robot2_wedge_lifter_option (Autodesk Fusion 360 design; units mm, degrees)
part number: 2026-09-22-20-04-37-960
part number: 2026-09-22-20-04-48-798
part number: 2026-09-22-20-04-48-802
part number: 2026-09-22-20-04-48-804
part number: 2026-09-22-20-04-48-807
part number: 2026-09-22-20-04-48-809
part number: 2026-09-22-20-10-09-073
part number: 2026-09-22-20-12-27-334
part number: 2026-09-22-20-12-27-362
part number: 2026-09-22-20-14-47-754
part number: 2026-09-22-20-14-47-792
part number: 2026-09-22-20-17-28-654
part number: 2026-09-22-20-20-38-193
part number: 2026-09-22-20-34-57-722
part number: 2026-09-22-20-34-57-795
part number: 2026-09-22-20-34-57-849
part number: 2026-09-22-20-34-57-901
part number: 2026-09-22-20-49-00-878
part number: 2026-09-22-20-49-00-891
part number: 2026-09-22-20-49-00-904
part number: 2026-09-22-20-50-05-757
part number: 2026-09-22-21-16-08-475
part number: 2026-09-22-21-16-09-075
part number: 2026-09-22-21-17-04-467
part number: 2026-09-22-21-17-04-732
part number: 2026-09-22-21-17-05-000
part number: 2026-09-22-21-17-05-645
part number: 2026-09-22-21-40-15-382
part number: 2026-09-22-21-42-45-679
part number: 2026-09-22-22-28-33-537
part number: 2026-09-22-22-50-56-103
part number: 2026-09-22-22-50-56-432
part number: 2026-09-22-22-50-56-745
part number: 2026-09-22-22-50-57-029
part number: 2026-09-22-23-22-03-101
part number: 2026-09-22-23-22-04-161
part number: 2026-09-22-23-22-05-011
part number: 2026-09-22-23-22-05-941
part number: 2026-09-22-23-30-32-609
part number: 2026-09-22-23-30-32-928
part number: 2026-09-22-23-34-46-416
part number: 2026-09-23-02-03-55-828
part number: 2026-09-23-02-03-56-507
part number: 2026-09-23-02-25-34-565
part number: 2026-09-23-02-25-35-125
part number: 2026-09-23-02-25-37-427
part number: 2026-09-23-02-25-38-082
part number: 2026-09-23-02-25-40-527
part number: 2026-09-23-02-25-41-161
part number: 2026-09-23-02-25-43-941
part number: 2026-09-23-02-25-44-578
part number: 2026-09-23-02-25-47-286
part number: 2026-09-23-02-25-47-976
part number: 2026-09-23-02-47-40-033
part number: 2026-09-23-02-47-40-739
part number: 2026-09-23-21-12-34-593
part number: 2026-09-23-21-12-34-998
part number: 2026-09-24-00-47-49-327
part number: 2026-09-24-00-47-50-049
part number: 2026-09-24-00-50-23-317
part number: 2026-09-24-00-50-23-446
part number: 2026-09-24-00-50-24-006
part number: 2026-09-24-00-50-24-800
part number: 2026-09-24-00-50-25-274
part number: 2026-09-24-00-50-26-431
part number: 2026-09-24-00-50-26-900
part number: 2026-09-24-00-50-27-361
part number: 2026-09-24-00-50-27-846
part number: 2026-09-24-00-55-06-014
part number: 2026-09-24-00-55-06-159
part number: 2026-09-24-00-55-06-686
part number: 2026-09-24-00-55-07-196
part number: 2026-09-24-00-55-07-718
part number: 2026-09-24-00-55-08-223
part number: 2026-09-24-00-55-08-760
part number: 2026-09-24-00-55-09-297
part number: 2026-09-24-00-55-09-817
Autodesk Fusion 360 part; units mm, degrees
note: some values were not read from the file. Chosen so that the rebuilt part matches the saved one: which bodies a step acts on.
(part 1 of 3)
sketch "Master_Layout_Top" plane through (0, 0, 0) normal (0, 0, 1) x (1, 0, 0)
  line L0 (80, 90) -> (-80, 90)
  line L1 (-80, 90) -> (-80, -90)
  line L2 (-80, -90) -> (80, -90)
  line L3 (80, -90) -> (80, 90)
  line L4 (0, -90) -> (0, 90) construction
  line L5 (-60.5714, 20.4286) -> (-79.5714, 20.4286)
  line L6 (-79.5714, 20.4286) -> (-79.5714, -21.5714)
  line L7 (-79.5714, -21.5714) -> (-60.5714, -21.5714)
  line L8 (-60.5714, -21.5714) -> (-60.5714, 20.4286)
  line L9 (79.4286, 20.4286) -> (60.4286, 20.4286)
  line L10 (60.4286, 20.4286) -> (60.4286, -21.5714)
  line L11 (60.4286, -21.5714) -> (79.4286, -21.5714)
  line L12 (79.4286, -21.5714) -> (79.4286, 20.4286)
  line L13 (25, -15) -> (-25, -15) construction
  line L14 (-25, -15) -> (-25, -75) construction
  line L15 (-25, -75) -> (25, -75) construction
  line L16 (25, -75) -> (25, -15) construction
  point P0 (0, 90)
  dimension "d14" = 160
  dimension "d15" = 180
  dimension "d16" = 19
  dimension "d17" = 42
  dimension "d18" = 19
  dimension "d19" = 42
  dimension "d20" = 50
  dimension "d21" = 60
  measures "d14" horizontal distance of L0.start L0.end
  measures "d15" vertical distance of L0.end L1.end
  measures "d16" horizontal distance of L5.start L5.end
  measures "d17" vertical distance of L5.end L6.end
  measures "d18" horizontal distance of L9.start L9.end
  measures "d19" vertical distance of L9.end L10.end
  measures "d20" horizontal distance of L13.start L13.end
  measures "d21" vertical distance of L13.end L14.end
sketch "Base_Plate_Sketch" plane through (0, 0, 0) normal (0, 0, 1) x (1, 0, 0) in component "Base_Plate_Al"
  line L0 (80, 90) -> (-80, 90)
  line L1 (-80, 90) -> (-80, -90)
  line L2 (-80, -90) -> (80, -90)
  line L3 (80, -90) -> (80, 90)
  dimension "d26" = 160
  dimension "d27" = 180
  measures "d26" horizontal distance of L0.start L0.end
  measures "d27" vertical distance of L0.end L1.end
extrude "Extrude1" add sketch "Base_Plate_Sketch" against normal blind 2 makes body 1 in component "Base_Plate_Al"
ref_plane "WorkPlane1" through (-80, 0, 0) normal (1, 0, 0) x (0, 1, 0) in component "Left_Side_Plate_Al"
sketch "Left_Plate_Sketch" plane through (-80, 0, 0) normal (1, 0, 0) x (0, 0, -1) in component "Left_Side_Plate_Al"
  line L0 (0, -90) -> (-78, -90)
  line L1 (-78, -90) -> (-78, 90)
  line L2 (-78, 90) -> (0, 90)
  line L3 (0, 90) -> (0, -90)
  dimension "d58" = 78
  dimension "d59" = 180
  measures "d58" horizontal distance of L0.start L0.end
  measures "d59" vertical distance of L0.end L1.end
extrude "Extrude1'" add sketch "Left_Plate_Sketch" along normal blind 2 separate body makes body 2 in component "Left_Side_Plate_Al"
ref_plane "WorkPlane1" through (80, 0, 0) normal (1, 0, 0) x (0, 1, 0) in component "Right_Side_Plate_Al"
sketch "Right_Plate_Sketch" plane through (80, 0, 0) normal (1, 0, 0) x (0, 0, -1) in component "Right_Side_Plate_Al"
  line L0 (0, -90) -> (-78, -90)
  line L1 (-78, -90) -> (-78, 90)
  line L2 (-78, 90) -> (0, 90)
  line L3 (0, 90) -> (0, -90)
  dimension "d64" = 78
  dimension "d65" = 180
  measures "d64" horizontal distance of L0.start L0.end
  measures "d65" vertical distance of L0.end L1.end
extrude "Extrude1''" add sketch "Right_Plate_Sketch" against normal blind 2 separate body makes body 3 in component "Right_Side_Plate_Al"
ref_plane "WorkPlane1" through (-80, 0, 0) normal (1, 0, 0) x (0, 1, 0) in component "Left_Wheel"
sketch "Left_Wheel_Sketch" plane through (-80, 0, 0) normal (1, 0, 0) x (0, 0, -1) in component "Left_Wheel"
  circle A0 centre (-21, 0) radius 21
  dimension "d70" = 42
  dimension "d208" = 21
  measures "d70" diameter of A0
  measures "d208" horizontal distance of origin A0.centre
extrude "Extrude1'''" add sketch "Left_Wheel_Sketch" along normal blind 19 separate body makes body 4 in component "Left_Wheel"
ref_plane "WorkPlane1" through (80, 0, 0) normal (1, 0, 0) x (0, 1, 0) in component "Right_Wheel"
sketch "Right_Wheel_Sketch" plane through (80, 0, 0) normal (1, 0, 0) x (0, 0, -1) in component "Right_Wheel"
  circle A0 centre (-21, 0) radius 21
  dimension "d75" = 42
  dimension "d209" = 21
  measures "d75" diameter of A0
  measures "d209" horizontal distance of origin A0.centre
extrude "Extrude1''''" add sketch "Right_Wheel_Sketch" against normal blind 19 separate body makes body 5 in component "Right_Wheel"
ref_plane "WorkPlane1" through (0, 0, 78) normal (0, 0, 1) x (1, 0, 0) in component "Top_Cover"
sketch "Top_Cover_Sketch" plane through (0, 0, 78) normal (0, 0, 1) x (1, 0, 0) in component "Top_Cover"
  line L0 (80, 90) -> (-80, 90)
  line L1 (-80, 90) -> (-80, -90)
  line L2 (-80, -90) -> (80, -90)
  line L3 (80, -90) -> (80, 90)
  dimension "d106" = 160
  dimension "d107" = 180
  measures "d106" horizontal distance of L0.start L0.end
  measures "d107" vertical distance of L0.end L1.end
extrude "Extrude1'''''" add sketch "Top_Cover_Sketch" along normal blind 2 separate body makes body 6 in component "Top_Cover"
sketch "Left_WedgeTrim_Sketch" plane through (-80, 0, 0) normal (1, 0, 0) x (0, 0, -1) in component "Left_Side_Plate_Al"
  line L0 (100, 40) -> (-100, 40)
  line L1 (-100, 40) -> (-100, 92)
  line L2 (-100, 92) -> (100, 92)
  line L3 (100, 92) -> (100, 40)
extrude "Extrude4" cut sketch "Left_WedgeTrim_Sketch" along normal mid plane 10 bodies 2 in component "Left_Side_Plate_Al"
sketch "Right_WedgeTrim_Sketch" plane through (80, 0, 0) normal (1, 0, 0) x (0, 0, -1) in component "Right_Side_Plate_Al"
  line L0 (100, 40) -> (-100, 40)
  line L1 (-100, 40) -> (-100, 92)
  line L2 (-100, 92) -> (100, 92)
  line L3 (100, 92) -> (100, 40)
extrude "Extrude4'" cut sketch "Right_WedgeTrim_Sketch" along normal mid plane 10 bodies 3 in component "Right_Side_Plate_Al"
sketch "Left_WheelWell_Sketch" plane through (-80, 0, 0) normal (1, 0, 0) x (0, 0, -1) in component "Left_Side_Plate_Al"
  line L0 (10, -26) -> (-42, -26)
  line L1 (-42, -26) -> (-42, 26)
  line L2 (-42, 26) -> (10, 26)
  line L3 (10, 26) -> (10, -26)
extrude "Extrude5" cut sketch "Left_WheelWell_Sketch" along normal mid plane 10 bodies 2 in component "Left_Side_Plate_Al"
sketch "Right_WheelWell_Sketch" plane through (80, 0, 0) normal (1, 0, 0) x (0, 0, -1) in component "Right_Side_Plate_Al"
  line L0 (10, -26) -> (-42, -26)
  line L1 (-42, -26) -> (-42, 26)
  line L2 (-42, 26) -> (10, 26)
  line L3 (10, 26) -> (10, -26)
extrude "Extrude5'" cut sketch "Right_WheelWell_Sketch" along normal mid plane 10 bodies 3 in component "Right_Side_Plate_Al"
ref_plane "WorkPlane1" through (-61, 0, 0) normal (1, 0, 0) x (0, 1, 0) in component "TT_Gearbox_L"
sketch "TT_Gearbox_L_Sketch" plane through (-61, 0, 0) normal (1, 0, 0) x (0, 0, -1) in component "TT_Gearbox_L"
  line L0 (-12, 11) -> (-30, 11)
  line L1 (-30, 11) -> (-30, -11)
  line L2 (-30, -11) -> (-12, -11)
  line L3 (-12, -11) -> (-12, 11)
  dimension "d228" = 18
  dimension "d229" = 22
  measures "d228" horizontal distance of L0.start L0.end
  measures "d229" vertical distance of L0.end L1.end
extrude "Extrude1''''''" add sketch "TT_Gearbox_L_Sketch" along normal blind 24 separate body makes body 7 in component "TT_Gearbox_L"
ref_plane "WorkPlane1" through (-3.7, 0, 0) normal (1, 0, 0) x (0, 1, 0) in component "TT_Motor_Can_L"
sketch "TT_Motor_Can_L_Sketch" plane through (-3.7, 0, 0) normal (1, 0, 0) x (0, 0, -1) in component "TT_Motor_Can_L"
  circle A0 centre (-21, 0) radius 10
  dimension "d234" = 20
  measures "d234" diameter of A0
extrude "Extrude2" add sketch "TT_Motor_Can_L_Sketch" against normal blind 25 separate body makes body 8 in component "TT_Motor_Can_L"
ref_plane "WorkPlane1" through (61, 0, 0) normal (1, 0, 0) x (0, 1, 0) in component "TT_Gearbox_R"
sketch "TT_Gearbox_R_Sketch" plane through (61, 0, 0) normal (1, 0, 0) x (0, 0, -1) in component "TT_Gearbox_R"
  line L0 (-12, 11) -> (-30, 11)
  line L1 (-30, 11) -> (-30, -11)
  line L2 (-30, -11) -> (-12, -11)
  line L3 (-12, -11) -> (-12, 11)
  dimension "d241" = 18
  dimension "d242" = 22
  measures "d241" horizontal distance of L0.start L0.end
  measures "d242" vertical distance of L0.end L1.end
extrude "Extrude1'''''''" add sketch "TT_Gearbox_R_Sketch" against normal blind 24 separate body makes body 9 in component "TT_Gearbox_R"
ref_plane "WorkPlane1" through (3.7, 0, 0) normal (1, 0, 0) x (0, 1, 0) in component "TT_Motor_Can_R"
sketch "TT_Motor_Can_R_Sketch" plane through (3.7, 0, 0) normal (1, 0, 0) x (0, 0, -1) in component "TT_Motor_Can_R"
  circle A0 centre (-21, 0) radius 10
  dimension "d247" = 20
  measures "d247" diameter of A0
extrude "Extrude2'" add sketch "TT_Motor_Can_R_Sketch" along normal blind 25 separate body makes body 10 in component "TT_Motor_Can_R"
ref_plane "WorkPlane1" through (0, 0, 31.6) normal (0, 0, 1) x (1, 0, 0) in component "Battery_and_Tray"
sketch "Battery_and_Tray_Sketch" plane through (0, 0, 31.6) normal (0, 0, 1) x (1, 0, 0) in component "Battery_and_Tray"
  line L0 (-52, -55.5) -> (52, -55.5)
  line L1 (52, -55.5) -> (52, -20.5)
  line L2 (52, -20.5) -> (-52, -20.5)
  line L3 (-52, -20.5) -> (-52, -55.5)
  dimension "d430" = 104
  dimension "d431" = 35
  measures "d430" horizontal distance of L0.start L0.end
  measures "d431" vertical distance of L0.end L1.end
extrude "Extrude1''''''''" add sketch "Battery_and_Tray_Sketch" along normal blind 27 separate body makes body 11 in component "Battery_and_Tray"
sketch "Left_Base_WheelCut_Sketch" plane through (0, 0, 0) normal (0, 0, 1) x (1, 0, 0) in component "Base_Plate_Al"
  line L0 (-90, -24) -> (-58, -24)
  line L1 (-58, -24) -> (-58, 24)
  line L2 (-58, 24) -> (-90, 24)
  line L3 (-90, 24) -> (-90, -24)
extrude "Extrude2''" cut sketch "Left_Base_WheelCut_Sketch" along normal mid plane 10 bodies 1 in component "Base_Plate_Al"
sketch "Right_Base_WheelCut_Sketch" plane through (0, 0, 0) normal (0, 0, 1) x (1, 0, 0) in component "Base_Plate_Al"
  line L0 (90, -24) -> (58, -24)
  line L1 (58, -24) -> (58, 24)
  line L2 (58, 24) -> (90, 24)
  line L3 (90, 24) -> (90, -24)
extrude "Extrude3" cut sketch "Right_Base_WheelCut_Sketch" along normal mid plane 10 bodies 1 in component "Base_Plate_Al"
move_body "GroundClearanceOffset" bodies 1 to x (1, 0, 0) y (0, 1, 0) z (0, 0, 1) at (0, 0, 5) in component "Base_Plate_Al"
move_body "GroundClearanceOffset'" bodies 2 to x (1, 0, 0) y (0, 1, 0) z (0, 0, 1) at (0, 0, 5) in component "Left_Side_Plate_Al"
move_body "GroundClearanceOffset''" bodies 3 to x (1, 0, 0) y (0, 1, 0) z (0, 0, 1) at (0, 0, 5) in component "Right_Side_Plate_Al"
move_body "GroundClearanceOffset'''" bodies 6 to x (1, 0, 0) y (0, 1, 0) z (0, 0, 1) at (0, 0, 5) in component "Top_Cover"
ref_plane "WorkPlane1" through (-80, 0, 0) normal (1, 0, 0) x (0, 1, 0) in component "Front_Wedge_L"
sketch "L_Wedge_Sketch" plane through (-80, 0, 0) normal (1, 0, 0) x (0, 0, -1) in component "Front_Wedge_L"
  line L0 (0, 90) -> (0, 40)
  line L1 (0, 40) -> (-78, 40)
  line L2 (-78, 40) -> (0, 90)
  dimension "d488" = 50
  dimension "d489" = 78
  dimension "d490" = 90
  measures "d488" vertical distance of L0.start L0.end
  measures "d489" horizontal distance of L0.end L1.end
  measures "d490" vertical distance of origin L0.start
extrude "Extrude1'''''''''" add sketch "L_Wedge_Sketch" along normal blind 45 separate body makes body 12 in component "Front_Wedge_L"
move_body "Move1" bodies 12 to x (1, 0, 0) y (0, 1, 0) z (0, 0, 1) at (0, 0, 5) in component "Front_Wedge_L"
ref_plane "WorkPlane1" through (80, 0, 0) normal (1, 0, 0) x (0, 1, 0) in component "Front_Wedge_R"
sketch "R_Wedge_Sketch" plane through (80, 0, 0) normal (1, 0, 0) x (0, 0, -1) in component "Front_Wedge_R"
  line L0 (0, 90) -> (0, 40)
  line L1 (0, 40) -> (-78, 40)
  line L2 (-78, 40) -> (0, 90)
  dimension "d498" = 50
  dimension "d499" = 78
  dimension "d500" = 90
  measures "d498" vertical distance of L0.start L0.end
  measures "d499" horizontal distance of L0.end L1.end
  measures "d500" vertical distance of origin L0.start
extrude "Extrude1''''''''''" add sketch "R_Wedge_Sketch" against normal blind 45 separate body makes body 13 in component "Front_Wedge_R"
move_body "Move1'" bodies 13 to x (1, 0, 0) y (0, 1, 0) z (0, 0, 1) at (0, 0, 5) in component "Front_Wedge_R"
ref_plane "WorkPlane1" through (-32.5, 0, 0) normal (1, 0, 0) x (0, 1, 0) in component "Spinner_Shaft"
sketch "Spinner_Shaft_Sketch" plane through (-32.5, 0, 0) normal (1, 0, 0) x (0, 0, -1) in component "Spinner_Shaft"
  circle A0 centre (-38.5, 75) radius 2
  dimension "d508" = 4
  measures "d508" diameter of A0
extrude "Extrude1'''''''''''" add sketch "Spinner_Shaft_Sketch" along normal blind 65 separate body makes body 14 in component "Spinner_Shaft"
ref_plane "WorkPlane1" through (-32.5, 0, 0) normal (1, 0, 0) x (0, 1, 0) in component "Left_Support"
sketch "Left_Support_Sketch" plane through (-32.5, 0, 0) normal (1, 0, 0) x (0, 0, -1) in component "Left_Support"
  circle A0 centre (-38.5, 75) radius 6.5
  dimension "d513" = 13
  measures "d513" diameter of A0
extrude "Extrude1''''''''''''" add sketch "Left_Support_Sketch" along normal blind 10 separate body makes body 15 in component "Left_Support"
ref_plane "WorkPlane1" through (32.5, 0, 0) normal (1, 0, 0) x (0, 1, 0) in component "Right_Support"
sketch "Right_Support_Sketch" plane through (32.5, 0, 0) normal (1, 0, 0) x (0, 0, -1) in component "Right_Support"
  circle A0 centre (-38.5, 75) radius 6.5
  dimension "d518" = 13
  measures "d518" diameter of A0
extrude "Extrude1'''''''''''''" add sketch "Right_Support_Sketch" against normal blind 10 separate body makes body 16 in component "Right_Support"
ref_plane "WorkPlane1" through (-15, 0, 0) normal (1, 0, 0) x (0, 1, 0) in component "Spinner_Motor"
sketch "Spinner_Motor_Sketch" plane through (-15, 0, 0) normal (1, 0, 0) x (0, 0, -1) in component "Spinner_Motor"
  circle A0 centre (-38.5, 25.75) radius 13.75
  dimension "d528" = 27.5
  measures "d528" diameter of A0
extrude "Extrude1''''''''''''''" add sketch "Spinner_Motor_Sketch" along normal blind 30 separate body makes body 17 in component "Spinner_Motor"
sketch "Standoff_Base_Sketch" plane through (0, 0, 0) normal (0, 0, 1) x (1, 0, 0) in component "Standoffs_Fasteners"
  circle A0 centre (-75, -85) radius 3
  circle A1 centre (-75, -85) radius 1.6
  circle A2 centre (75, -85) radius 3
  circle A3 centre (75, -85) radius 1.6
  circle A4 centre (-75, 35) radius 3
  circle A5 centre (-75, 35) radius 1.6
  circle A6 centre (75, 35) radius 3
  circle A7 centre (75, 35) radius 1.6
  dimension "d563" = 6
  dimension "d564" = 3.2
  dimension "d565" = 6
  dimension "d566" = 3.2
  dimension "d567" = 6
  dimension "d568" = 3.2
  dimension "d569" = 6
  dimension "d570" = 3.2
  measures "d563" diameter of A0
  measures "d564" diameter of A1
  measures "d565" diameter of A2
  measures "d566" diameter of A3
  measures "d567" diameter of A4
  measures "d568" diameter of A5
  measures "d569" diameter of A6
  measures "d570" diameter of A7
extrude "Extrude1'''''''''''''''" add sketch "Standoff_Base_Sketch" along normal blind 78 from surface at 5 separate body contours A0 | A1 | A2 | A3 | A4 | A5 | A6 | A7 makes body 18 at (-76.3686, 32.3304, 31) makes body 19 at (72.3653, -86.4348, 57) makes body 20 at (-77.6347, -86.4348, 57) makes body 21 at (73.6314, 32.3304, 31) in component "Standoffs_Fasteners"
sketch "Base_Plate_Al_FastenerHoles" plane through (0, 0, 0) normal (0, 0, 1) x (1, 0, 0) in component "Base_Plate_Al"
  circle A0 centre (-75, -85) radius 1.7
  circle A1 centre (75, -85) radius 1.7
  circle A2 centre (-75, 35) radius 1.7
  circle A3 centre (75, 35) radius 1.7
extrude "Extrude4''" cut sketch "Base_Plate_Al_FastenerHoles" along normal mid plane 8 bodies 1 in component "Base_Plate_Al"
sketch "Top_Cover_FastenerHoles" plane through (0, 0, 0) normal (0, 0, 1) x (1, 0, 0) in component "Top_Cover"
  circle A0 centre (-75, -85) radius 1.7
  circle A1 centre (75, -85) radius 1.7
  circle A2 centre (-75, 35) radius 1.7
  circle A3 centre (75, 35) radius 1.7
extrude "Extrude2'''" cut sketch "Top_Cover_FastenerHoles" along normal mid plane 8 bodies 6 in component "Top_Cover"
sketch "Left_FastenerHoles_Sketch" plane through (-80, 0, 0) normal (1, 0, 0) x (0, 0, -1) in component "Left_Side_Plate_Al"
  circle A0 centre (-44, -85) radius 1.7
  circle A1 centre (-44, 35) radius 1.7
extrude "Extrude6" cut sketch "Left_FastenerHoles_Sketch" along normal mid plane 10 bodies 2 in component "Left_Side_Plate_Al"
sketch "Right_FastenerHoles_Sketch" plane through (80, 0, 0) normal (1, 0, 0) x (0, 0, -1) in component "Right_Side_Plate_Al"
  circle A0 centre (-44, -85) radius 1.7
  circle A1 centre (-44, 35) radius 1.7
extrude "Extrude6'" cut sketch "Right_FastenerHoles_Sketch" along normal mid plane 10 bodies 3 in component "Right_Side_Plate_Al"
sketch "L_TT_MountHoles" plane through (-61, 0, 0) normal (1, 0, 0) x (0, 0, -1) in component "TT_Gearbox_L"
  circle A0 centre (-21, -8.75) radius 1.7
  circle A1 centre (-21, 8.75) radius 1.7
extrude "Extrude2''''" cut sketch "L_TT_MountHoles" along normal mid plane 72 bodies 7 in component "TT_Gearbox_L"
sketch "R_TT_MountHoles" plane through (61, 0, 0) normal (1, 0, 0) x (0, 0, -1) in component "TT_Gearbox_R"
  circle A0 centre (-21, -8.75) radius 1.7
  circle A1 centre (-21, 8.75) radius 1.7
extrude "Extrude2'''''" cut sketch "R_TT_MountHoles" along normal mid plane 72 bodies 9 in component "TT_Gearbox_R"
sketch "Spinner_Motor_MountHoles" plane through (-15, 0, 0) normal (1, 0, 0) x (0, 0, -1) in component "Spinner_Motor"
  circle A0 centre (-8, -9.5) radius 1.7
  circle A1 centre (-8, 9.5) radius 1.7
  circle A2 centre (8, -9.5) radius 1.7
  circle A3 centre (8, 9.5) radius 1.7
extrude "Extrude2''''''" cut sketch "Spinner_Motor_MountHoles" along normal mid plane 90 bodies 17 in component "Spinner_Motor"
sketch "Servo_FlangeHoles" plane through (0, 0, 0) normal (0, 0, 1) x (1, 0, 0) in component "Top_Cover"
  circle A0 centre (0, -24.75) radius 1.7
  circle A1 centre (0, 24.75) radius 1.7
extrude "Extrude3'" cut sketch "Servo_FlangeHoles" along normal mid plane 8 bodies 6 in component "Top_Cover"
ref_plane "WorkPlane1" through (0, 0, 29.6) normal (0, 0, 1) x (1, 0, 0) in component "Battery_Holder"
sketch "Holder_Floor_Sketch" plane through (0, 0, 29.6) normal (0, 0, 1) x (1, 0, 0) in component "Battery_Holder"
  line L0 (-52, -55.5) -> (52, -55.5)
  line L1 (52, -55.5) -> (52, -20.5)
  line L2 (52, -20.5) -> (-52, -20.5)
  line L3 (-52, -20.5) -> (-52, -55.5)
  dimension "d597" = 104
  dimension "d598" = 35
  measures "d597" horizontal distance of L0.start L0.end
  measures "d598" vertical distance of L0.end L1.end
extrude "Extrude1''''''''''''''''" add sketch "Holder_Floor_Sketch" along normal blind 2 separate body makes body 22 in component "Battery_Holder"
sketch "Holder_StrapSlots" plane through (0, 0, 29.6) normal (0, 0, 1) x (1, 0, 0) in component "Battery_Holder"
  line L0 (-39, -43) -> (-35, -43)
  line L1 (-35, -43) -> (-35, -33)
  line L2 (-35, -33) -> (-39, -33)
  line L3 (-39, -33) -> (-39, -43)
  line L4 (35, -43) -> (39, -43)
  line L5 (39, -43) -> (39, -33)
  line L6 (39, -33) -> (35, -33)
  line L7 (35, -33) -> (35, -43)
extrude "Extrude2'''''''" cut sketch "Holder_StrapSlots" along normal mid plane 10 bodies 22 in component "Battery_Holder"
ref_plane "WorkPlane2" through (0, 0, 31.6) normal (0, 0, 1) x (1, 0, 0) in component "Battery_Holder"
sketch "Sketch3" plane through (0, 0, 31.6) normal (0, 0, 1) x (1, 0, 0) in component "Battery_Holder"
  line L0 (-52, -57.5) -> (52, -57.5)
  line L1 (52, -57.5) -> (52, -55.5)
  line L2 (52, -55.5) -> (-52, -55.5)
  line L3 (-52, -55.5) -> (-52, -57.5)
extrude "Extrude3''" add sketch "Sketch3" along normal blind 5 bodies 22 in component "Battery_Holder"
sketch "Sketch4" plane through (0, 0, 31.6) normal (0, 0, 1) x (1, 0, 0) in component "Battery_Holder"
  line L0 (-52, -20.5) -> (52, -20.5)
  line L1 (52, -20.5) -> (52, -18.5)
  line L2 (52, -18.5) -> (-52, -18.5)
  line L3 (-52, -18.5) -> (-52, -20.5)
extrude "Extrude4'''" add sketch "Sketch4" along normal blind 5 bodies 22 in component "Battery_Holder"
move_body "Move1''" bodies 22 to x (1, 0, 0) y (0, 1, 0) z (0, 0, 1) at (0, 0, 3) in component "Battery_Holder"
move_body "Move1'''" bodies 11 to x (1, 0, 0) y (0, 1, 0) z (0, 0, 1) at (0, 0, 3) in component "Battery_and_Tray"
sketch "L_Wedge_ScrewHoles" plane through (0, 0, 0) normal (0, 0, 1) x (1, 0, 0) in component "Front_Wedge_L"
  circle A0 centre (-73, 80) radius 1.7
  circle A1 centre (-50, 50) radius 1.7
extrude "Extrude2''''''''" cut sketch "L_Wedge_ScrewHoles" along normal mid plane 12 bodies 12 in component "Front_Wedge_L"
sketch "L_WedgeScrew_BaseHoles" plane through (0, 0, 0) normal (0, 0, 1) x (1, 0, 0) in component "Base_Plate_Al"
  circle A0 centre (-73, 80) radius 1.7
  circle A1 centre (-50, 50) radius 1.7
extrude "Extrude6''" cut sketch "L_WedgeScrew_BaseHoles" along normal mid plane 12 bodies 1 in component "Base_Plate_Al"
sketch "R_Wedge_ScrewHoles" plane through (0, 0, 0) normal (0, 0, 1) x (1, 0, 0) in component "Front_Wedge_R"
  circle A0 centre (73, 80) radius 1.7
  circle A1 centre (50, 50) radius 1.7
extrude "Extrude2'''''''''" cut sketch "R_Wedge_ScrewHoles" along normal mid plane 12 bodies 13 in component "Front_Wedge_R"
sketch "R_WedgeScrew_BaseHoles" plane through (0, 0, 0) normal (0, 0, 1) x (1, 0, 0) in component "Base_Plate_Al"
  circle A0 centre (73, 80) radius 1.7
  circle A1 centre (50, 50) radius 1.7
extrude "Extrude7" cut sketch "R_WedgeScrew_BaseHoles" along normal mid plane 12 bodies 1 in component "Base_Plate_Al"
sketch "Left_TT_MountHoles" plane through (-80, 0, 0) normal (1, 0, 0) x (0, 0, -1) in component "Left_Side_Plate_Al"
  circle A0 centre (-21, -8.75) radius 1.7
  circle A1 centre (-21, 8.75) radius 1.7
extrude "Extrude7'" cut sketch "Left_TT_MountHoles" along normal mid plane 12 bodies 2 in component "Left_Side_Plate_Al"
sketch "Right_TT_MountHoles" plane through (80, 0, 0) normal (1, 0, 0) x (0, 0, -1) in component "Right_Side_Plate_Al"
  circle A0 centre (-21, -8.75) radius 1.7
  circle A1 centre (-21, 8.75) radius 1.7
extrude "Extrude7''" cut sketch "Right_TT_MountHoles" along normal mid plane 12 bodies 3 in component "Right_Side_Plate_Al"
sketch "RollPin_Hole" plane through (0, 0, 0) normal (0, 0, 1) x (1, 0, 0) in component "Spinner_Shaft"
  circle A0 centre (0, 75) radius 1
extrude "Extrude2''''''''''" cut sketch "RollPin_Hole" along normal mid plane 60 bodies 14 in component "Spinner_Shaft"
sketch "Cradle_Block_Sketch" plane through (0, 0, 0) normal (0, 0, 1) x (1, 0, 0) in component "Spinner_Motor_Cradle"
  line L0 (-15, 12) -> (15, 12)
  line L1 (15, 12) -> (15, 41)
  line L2 (15, 41) -> (-15, 41)
  line L3 (-15, 41) -> (-15, 12)
extrude "Extrude1'''''''''''''''''" add sketch "Cradle_Block_Sketch" along normal blind 25.5 from surface at 5 separate body makes body 23 in component "Spinner_Motor_Cradle"
sketch "Cradle_Saddle_Sketch" plane through (0, 0, 0) normal (1, 0, 0) x (0, 0, -1) in component "Spinner_Motor_Cradle"
  circle A0 centre (-38.5, 25.75) radius 14.15
extrude "Extrude2'''''''''''" cut sketch "Cradle_Saddle_Sketch" along normal mid plane 50 bodies 23 in component "Spinner_Motor_Cradle"
sketch "Cradle_Bolt_Sketch" plane through (0, 0, 0) normal (0, 0, 1) x (1, 0, 0) in component "Spinner_Motor_Cradle"
  circle A0 centre (-11, 16) radius 1.25
  circle A1 centre (11, 16) radius 1.25
  circle A2 centre (-11, 37) radius 1.25
  circle A3 centre (11, 37) radius 1.25
extrude "Extrude3'''" cut sketch "Cradle_Bolt_Sketch" along normal blind 8 from surface at 5 bodies 23 in component "Spinner_Motor_Cradle"
sketch "Cradle_Bolt_Clearance_Sketch" plane through (0, 0, 0) normal (0, 0, 1) x (1, 0, 0) in component "Base_Plate_Al"
  circle A0 centre (-11, 16) radius 1.7
  circle A1 centre (11, 16) radius 1.7
  circle A2 centre (-11, 37) radius 1.7
  circle A3 centre (11, 37) radius 1.7
extrude "Extrude8" cut sketch "Cradle_Bolt_Clearance_Sketch" along normal mid plane 30 bodies 1 in component "Base_Plate_Al"
sketch "TT_Mount_Clearance_Sketch_L" plane through (0, 0, 0) normal (0, 0, 1) x (1, 0, 0) in component "Base_Plate_Al"
  circle A0 centre (-51, -14) radius 1.7
  circle A1 centre (-51, 14) radius 1.7
  circle A2 centre (-38.7, -14) radius 1.7
  circle A3 centre (-38.7, 14) radius 1.7
extrude "Extrude10" cut sketch "TT_Mount_Clearance_Sketch_L" along normal mid plane 30 bodies 1 in component "Base_Plate_Al"
sketch "TT_Mount_Clearance_Sketch_R" plane through (0, 0, 0) normal (0, 0, 1) x (1, 0, 0) in component "Base_Plate_Al"
  circle A0 centre (38.7, -14) radius 1.7
  circle A1 centre (38.7, 14) radius 1.7
  circle A2 centre (51, -14) radius 1.7
  circle A3 centre (51, 14) radius 1.7
extrude "Extrude11" cut sketch "TT_Mount_Clearance_Sketch_R" along normal mid plane 30 bodies 1 in component "Base_Plate_Al"
sketch "TT_Mount_Block_Sketch" plane through (0, 0, 0) normal (0, 0, 1) x (1, 0, 0) in component "TT_Motor_Mount_L"
  line L0 (-55, -16.5) -> (-34.7, -16.5)
  line L1 (-34.7, -16.5) -> (-34.7, 16.5)
  line L2 (-34.7, 16.5) -> (-55, 16.5)
  line L3 (-55, 16.5) -> (-55, -16.5)
extrude "Extrude1''''''''''''''''''" add sketch "TT_Mount_Block_Sketch" along normal blind 23.5 from surface at 5 separate body makes body 24 in component "TT_Motor_Mount_L"
sketch "TT_Mount_Pocket_Sketch" plane through (0, 0, 0) normal (0, 0, 1) x (1, 0, 0) in component "TT_Motor_Mount_L"
  line L0 (-60, -11.5) -> (-29.7, -11.5)
  line L1 (-29.7, -11.5) -> (-29.7, 11.5)
  line L2 (-29.7, 11.5) -> (-60, 11.5)
  line L3 (-60, 11.5) -> (-60, -11.5)
extrude "Extrude2''''''''''''" cut sketch "TT_Mount_Pocket_Sketch" along normal blind 26.5 from surface at 12 bodies 24 in component "TT_Motor_Mount_L"
sketch "TT_Mount_Bolt_Sketch" plane through (0, 0, 0) normal (0, 0, 1) x (1, 0, 0) in component "TT_Motor_Mount_L"
  circle A0 centre (-51, -14) radius 1.25
  circle A1 centre (-51, 14) radius 1.25
  circle A2 centre (-38.7, -14) radius 1.25
  circle A3 centre (-38.7, 14) radius 1.25
extrude "Extrude3''''" cut sketch "TT_Mount_Bolt_Sketch" along normal blind 5 from surface at 5 bodies 24 in component "TT_Motor_Mount_L"
sketch "TT_Mount_ClampTap_Sketch" plane through (0, 0, 0) normal (0, 0, 1) x (1, 0, 0) in component "TT_Motor_Mount_L"
  circle A0 centre (-44.85, -14) radius 1.25
  circle A1 centre (-44.85, 14) radius 1.25
extrude "Extrude4''''" cut sketch "TT_Mount_ClampTap_Sketch" against normal blind 8 from surface at 28.5 bodies 24 in component "TT_Motor_Mount_L"
sketch "TT_Clamp_Sketch" plane through (0, 0, 0) normal (0, 0, 1) x (1, 0, 0) in component "TT_Motor_Clamp_L"
  line L0 (-49.85, -16.5) -> (-39.85, -16.5)
  line L1 (-39.85, -16.5) -> (-39.85, 16.5)
  line L2 (-39.85, 16.5) -> (-49.85, 16.5)
  line L3 (-49.85, 16.5) -> (-49.85, -16.5)
extrude "Extrude1'''''''''''''''''''" add sketch "TT_Clamp_Sketch" along normal blind 3 from surface at 30 separate body makes body 25 in component "TT_Motor_Clamp_L"
sketch "TT_Clamp_Holes_Sketch" plane through (0, 0, 0) normal (0, 0, 1) x (1, 0, 0) in component "TT_Motor_Clamp_L"
  circle A0 centre (-44.85, -14) radius 1.7
  circle A1 centre (-44.85, 14) radius 1.7
extrude "Extrude2'''''''''''''" cut sketch "TT_Clamp_Holes_Sketch" along normal mid plane 200 bodies 25 in component "TT_Motor_Clamp_L"
sketch "TT_Mount_Block_Sketch (2)" plane through (0, 0, 0) normal (0, 0, 1) x (1, 0, 0) in component "TT_Motor_Mount_R"
  line L0 (34.7, -16.5) -> (55, -16.5)
  line L1 (55, -16.5) -> (55, 16.5)
  line L2 (55, 16.5) -> (34.7, 16.5)
  line L3 (34.7, 16.5) -> (34.7, -16.5)
extrude "Extrude1''''''''''''''''''''" add sketch "TT_Mount_Block_Sketch (2)" along normal blind 23.5 from surface at 5 separate body makes body 26 in component "TT_Motor_Mount_R"
sketch "TT_Mount_Pocket_Sketch (2)" plane through (0, 0, 0) normal (0, 0, 1) x (1, 0, 0) in component "TT_Motor_Mount_R"
  line L0 (29.7, -11.5) -> (60, -11.5)
  line L1 (60, -11.5) -> (60, 11.5)
  line L2 (60, 11.5) -> (29.7, 11.5)
  line L3 (29.7, 11.5) -> (29.7, -11.5)
extrude "Extrude2''''''''''''''" cut sketch "TT_Mount_Pocket_Sketch (2)" along normal blind 26.5 from surface at 12 bodies 26 in component "TT_Motor_Mount_R"
sketch "TT_Mount_Bolt_Sketch (2)" plane through (0, 0, 0) normal (0, 0, 1) x (1, 0, 0) in component "TT_Motor_Mount_R"
  circle A0 centre (38.7, -14) radius 1.25
  circle A1 centre (38.7, 14) radius 1.25
  circle A2 centre (51, -14) radius 1.25
  circle A3 centre (51, 14) radius 1.25
extrude "Extrude3'''''" cut sketch "TT_Mount_Bolt_Sketch (2)" along normal blind 5 from surface at 5 bodies 26 in component "TT_Motor_Mount_R"
sketch "TT_Mount_ClampTap_Sketch (2)" plane through (0, 0, 0) normal (0, 0, 1) x (1, 0, 0) in component "TT_Motor_Mount_R"
  circle A0 centre (44.85, -14) radius 1.25
  circle A1 centre (44.85, 14) radius 1.25
extrude "Extrude4'''''" cut sketch "TT_Mount_ClampTap_Sketch (2)" against normal blind 8 from surface at 28.5 bodies 26 in component "TT_Motor_Mount_R"
sketch "TT_Clamp_Sketch (2)" plane through (0, 0, 0) normal (0, 0, 1) x (1, 0, 0) in component "TT_Motor_Clamp_R"
  line L0 (39.85, -16.5) -> (49.85, -16.5)
  line L1 (49.85, -16.5) -> (49.85, 16.5)
  line L2 (49.85, 16.5) -> (39.85, 16.5)
  line L3 (39.85, 16.5) -> (39.85, -16.5)
extrude "Extrude1'''''''''''''''''''''" add sketch "TT_Clamp_Sketch (2)" along normal blind 3 from surface at 30 separate body makes body 27 in component "TT_Motor_Clamp_R"
sketch "TT_Clamp_Holes_Sketch (2)" plane through (0, 0, 0) normal (0, 0, 1) x (1, 0, 0) in component "TT_Motor_Clamp_R"
  circle A0 centre (44.85, -14) radius 1.7
  circle A1 centre (44.85, 14) radius 1.7
extrude "Extrude2'''''''''''''''" cut sketch "TT_Clamp_Holes_Sketch (2)" along normal mid plane 200 bodies 27 in component "TT_Motor_Clamp_R"
sketch "Cover_Fastener_Holes" plane through (0, 0, 0) normal (0, 0, 1) x (1, 0, 0) in component "Top_Cover"
  circle A0 centre (-75, 35) radius 1.7
  circle A1 centre (75, -85) radius 1.7
  circle A2 centre (-75, -85) radius 1.7
  circle A3 centre (75, 35) radius 1.7
  circle A4 centre (0, 24.75) radius 1.7
  circle A5 centre (0, -24.75) radius 1.7
extrude "Extrude4''''''" cut sketch "Cover_Fastener_Holes" along normal blind 6 from surface at 81 bodies 6 in component "Top_Cover"
sketch "Corner_Standoff_Clearance" plane through (0, 0, 0) normal (0, 0, 1) x (1, 0, 0) in component "Base_Plate_Al"
  circle A0 centre (-75, 35) radius 1.7
  circle A1 centre (75, -85) radius 1.7
  circle A2 centre (-75, -85) radius 1.7
  circle A3 centre (75, 35) radius 1.7
extrude "Extrude12" cut sketch "Corner_Standoff_Clearance" along normal blind 6 from surface at 1 bodies 1 in component "Base_Plate_Al"
sketch "Tap_Bottom" plane through (0, 0, 0) normal (0, 0, 1) x (1, 0, 0) in component "Standoffs_Fasteners"
  circle A0 centre (-75, 35) radius 1.25
extrude "Extrude2''''''''''''''''" cut sketch "Tap_Bottom" along normal blind 10 from surface at 5 bodies 18 in component "Standoffs_Fasteners"
sketch "Tap_Top" plane through (0, 0, 0) normal (0, 0, 1) x (1, 0, 0) in component "Standoffs_Fasteners"
  circle A0 centre (-75, 35) radius 1.25
extrude "Extrude3''''''" cut sketch "Tap_Top" against normal blind 10 from surface at 83 bodies 18 in component "Standoffs_Fasteners"
sketch "Tap_Side" plane through (0, 0, 0) normal (1, 0, 0) x (0, 0, -1) in component "Standoffs_Fasteners"
  circle A0 centre (-44, 35) radius 1.25
extrude "Extrude4'''''''" cut sketch "Tap_Side" along normal mid plane 400 bodies 18 in component "Standoffs_Fasteners"
sketch "Tap_Bottom_Standoff_2" plane through (0, 0, 0) normal (0, 0, 1) x (1, 0, 0) in component "Standoffs_Fasteners"
  circle A0 centre (75, -85) radius 1.25
extrude "Extrude5''" cut sketch "Tap_Bottom_Standoff_2" along normal blind 10 from surface at 5 bodies 19 in component "Standoffs_Fasteners"
sketch "Tap_Top_Standoff_2" plane through (0, 0, 0) normal (0, 0, 1) x (1, 0, 0) in component "Standoffs_Fasteners"
  circle A0 centre (75, -85) radius 1.25
extrude "Extrude6'''" cut sketch "Tap_Top_Standoff_2" against normal blind 10 from surface at 83 bodies 19 in component "Standoffs_Fasteners"
sketch "Tap_Side_Standoff_2" plane through (0, 0, 0) normal (1, 0, 0) x (0, 0, -1) in component "Standoffs_Fasteners"
  circle A0 centre (-44, -85) radius 1.25
extrude "Extrude7'''" cut sketch "Tap_Side_Standoff_2" along normal mid plane 400 bodies 19 in component "Standoffs_Fasteners"
sketch "Tap_Bottom_Standoff_3" plane through (0, 0, 0) normal (0, 0, 1) x (1, 0, 0) in component "Standoffs_Fasteners"
  circle A0 centre (-75, -85) radius 1.25
extrude "Extrude8'" cut sketch "Tap_Bottom_Standoff_3" along normal blind 10 from surface at 5 bodies 20 in component "Standoffs_Fasteners"
sketch "Tap_Top_Standoff_3" plane through (0, 0, 0) normal (0, 0, 1) x (1, 0, 0) in component "Standoffs_Fasteners"
  circle A0 centre (-75, -85) radius 1.25
extrude "Extrude9" cut sketch "Tap_Top_Standoff_3" against normal blind 10 from surface at 83 bodies 20 in component "Standoffs_Fasteners"
sketch "Tap_Side_Standoff_3" plane through (0, 0, 0) normal (1, 0, 0) x (0, 0, -1) in component "Standoffs_Fasteners"
  circle A0 centre (-44, -85) radius 1.25
extrude "Extrude10'" cut sketch "Tap_Side_Standoff_3" along normal mid plane 400 bodies 20 in component "Standoffs_Fasteners"
sketch "Tap_Bottom_Standoff_4" plane through (0, 0, 0) normal (0, 0, 1) x (1, 0, 0) in component "Standoffs_Fasteners"
  circle A0 centre (75, 35) radius 1.25
extrude "Extrude11'" cut sketch "Tap_Bottom_Standoff_4" along normal blind 10 from surface at 5 bodies 21 in component "Standoffs_Fasteners"
sketch "Tap_Top_Standoff_4" plane through (0, 0, 0) normal (0, 0, 1) x (1, 0, 0) in component "Standoffs_Fasteners"
  circle A0 centre (75, 35) radius 1.25
extrude "Extrude12'" cut sketch "Tap_Top_Standoff_4" against normal blind 10 from surface at 83 bodies 21 in component "Standoffs_Fasteners"
sketch "Tap_Side_Standoff_4" plane through (0, 0, 0) normal (1, 0, 0) x (0, 0, -1) in component "Standoffs_Fasteners"
  circle A0 centre (-44, 35) radius 1.25
extrude "Extrude13" cut sketch "Tap_Side_Standoff_4" along normal mid plane 400 bodies 21 in component "Standoffs_Fasteners"
sketch "Cradle_Lightening" plane through (0, 0, 0) normal (0, 1, 0) x (1, 0, 0) in component "Spinner_Motor_Cradle"
  line L0 (-9, -8) -> (9, -8)
  line L1 (9, -8) -> (9, -19)
  line L2 (9, -19) -> (-9, -19)
  line L3 (-9, -19) -> (-9, -8)
extrude "Extrude4''''''''" cut sketch "Cradle_Lightening" along normal mid plane 400 bodies 23 in component "Spinner_Motor_Cradle"
sketch "TT_Light_A_L" plane through (0, 0, 0) normal (0, 1, 0) x (1, 0, 0) in component "TT_Motor_Mount_L"
  line L0 (-53.5, -15.5) -> (-47.5, -15.5)
  line L1 (-47.5, -15.5) -> (-47.5, -26)
  line L2 (-47.5, -26) -> (-53.5, -26)
  line L3 (-53.5, -26) -> (-53.5, -15.5)
extrude "Extrude5'''" cut sketch "TT_Light_A_L" along normal mid plane 400 bodies 24 in component "TT_Motor_Mount_L"
sketch "TT_Light_B_L" plane through (0, 0, 0) normal (0, 1, 0) x (1, 0, 0) in component "TT_Motor_Mount_L"
  line L0 (-42.2, -15.5) -> (-36.2, -15.5)
  line L1 (-36.2, -15.5) -> (-36.2, -26)
  line L2 (-36.2, -26) -> (-42.2, -26)
  line L3 (-42.2, -26) -> (-42.2, -15.5)
extrude "Extrude6''''" cut sketch "TT_Light_B_L" along normal mid plane 400 bodies 24 in component "TT_Motor_Mount_L"
sketch "TT_Light_A_R" plane through (0, 0, 0) normal (0, 1, 0) x (1, 0, 0) in component "TT_Motor_Mount_R"
  line L0 (36.2, -15.5) -> (42.2, -15.5)
  line L1 (42.2, -15.5) -> (42.2, -26)
  line L2 (42.2, -26) -> (36.2, -26)
  line L3 (36.2, -26) -> (36.2, -15.5)
extrude "Extrude5''''" cut sketch "TT_Light_A_R" along normal mid plane 400 bodies 26 in component "TT_Motor_Mount_R"
sketch "TT_Light_B_R" plane through (0, 0, 0) normal (0, 1, 0) x (1, 0, 0) in component "TT_Motor_Mount_R"
  line L0 (47.5, -15.5) -> (53.5, -15.5)
  line L1 (53.5, -15.5) -> (53.5, -26)
  line L2 (53.5, -26) -> (47.5, -26)
  line L3 (47.5, -26) -> (47.5, -15.5)
extrude "Extrude6'''''" cut sketch "TT_Light_B_R" along normal mid plane 400 bodies 26 in component "TT_Motor_Mount_R"
sketch "Batt_Post_1_Sketch" plane through (0, 0, 0) normal (0, 0, 1) x (1, 0, 0) in component "Batt_Post_1"
  circle A0 centre (-34, -30) radius 2.5
extrude "Extrude1''''''''''''''''''''''" add sketch "Batt_Post_1_Sketch" along normal blind 27.6 from surface at 5 separate body makes body 28 in component "Batt_Post_1"
sketch "PilotTop_Batt_Post_1" plane through (0, 0, 0) normal (0, 0, 1) x (1, 0, 0) in component "Batt_Post_1"
  circle A0 centre (-34, -30) radius 1.05
extrude "Extrude2'''''''''''''''''" cut sketch "PilotTop_Batt_Post_1" against normal blind 8 from surface at 32.6 bodies 28 in component "Batt_Post_1"
sketch "PilotBot_Batt_Post_1" plane through (0, 0, 0) normal (0, 0, 1) x (1, 0, 0) in component "Batt_Post_1"
  circle A0 centre (-34, -30) radius 1.05
extrude "Extrude3'''''''" cut sketch "PilotBot_Batt_Post_1" along normal blind 8 from surface at 5 bodies 28 in component "Batt_Post_1"
sketch "Batt_Post_2_Sketch" plane through (0, 0, 0) normal (0, 0, 1) x (1, 0, 0) in component "Batt_Post_2"
  circle A0 centre (34, -30) radius 2.5
extrude "Extrude1'''''''''''''''''''''''" add sketch "Batt_Post_2_Sketch" along normal blind 27.6 from surface at 5 separate body makes body 29 in component "Batt_Post_2"
sketch "PilotTop_Batt_Post_2" plane through (0, 0, 0) normal (0, 0, 1) x (1, 0, 0) in component "Batt_Post_2"
  circle A0 centre (34, -30) radius 1.05
extrude "Extrude2''''''''''''''''''" cut sketch "PilotTop_Batt_Post_2" against normal blind 8 from surface at 32.6 bodies 29 in component "Batt_Post_2"
sketch "PilotBot_Batt_Post_2" plane through (0, 0, 0) normal (0, 0, 1) x (1, 0, 0) in component "Batt_Post_2"
  circle A0 centre (34, -30) radius 1.05
extrude "Extrude3''''''''" cut sketch "PilotBot_Batt_Post_2" along normal blind 8 from surface at 5 bodies 29 in component "Batt_Post_2"
sketch "Batt_Post_3_Sketch" plane through (0, 0, 0) normal (0, 0, 1) x (1, 0, 0) in component "Batt_Post_3"
  circle A0 centre (-34, -46) radius 2.5
extrude "Extrude1''''''''''''''''''''''''" add sketch "Batt_Post_3_Sketch" along normal blind 27.6 from surface at 5 separate body makes body 30 in component "Batt_Post_3"
sketch "PilotTop_Batt_Post_3" plane through (0, 0, 0) normal (0, 0, 1) x (1, 0, 0) in component "Batt_Post_3"
  circle A0 centre (-34, -46) radius 1.05
extrude "Extrude2'''''''''''''''''''" cut sketch "PilotTop_Batt_Post_3" against normal blind 8 from surface at 32.6 bodies 30 in component "Batt_Post_3"
sketch "PilotBot_Batt_Post_3" plane through (0, 0, 0) normal (0, 0, 1) x (1, 0, 0) in component "Batt_Post_3"
  circle A0 centre (-34, -46) radius 1.05
extrude "Extrude3'''''''''" cut sketch "PilotBot_Batt_Post_3" along normal blind 8 from surface at 5 bodies 30 in component "Batt_Post_3"
sketch "Batt_Post_4_Sketch" plane through (0, 0, 0) normal (0, 0, 1) x (1, 0, 0) in component "Batt_Post_4"
  circle A0 centre (34, -46) radius 2.5
extrude "Extrude1'''''''''''''''''''''''''" add sketch "Batt_Post_4_Sketch" along normal blind 27.6 from surface at 5 separate body makes body 31 in component "Batt_Post_4"
sketch "PilotTop_Batt_Post_4" plane through (0, 0, 0) normal (0, 0, 1) x (1, 0, 0) in component "Batt_Post_4"
  circle A0 centre (34, -46) radius 1.05
extrude "Extrude2''''''''''''''''''''" cut sketch "PilotTop_Batt_Post_4" against normal blind 8 from surface at 32.6 bodies 31 in component "Batt_Post_4"
sketch "PilotBot_Batt_Post_4" plane through (0, 0, 0) normal (0, 0, 1) x (1, 0, 0) in component "Batt_Post_4"
  circle A0 centre (34, -46) radius 1.05
extrude "Extrude3''''''''''" cut sketch "PilotBot_Batt_Post_4" along normal blind 8 from surface at 5 bodies 31 in component "Batt_Post_4"
sketch "Holder_Mount_Holes" plane through (0, 0, 0) normal (0, 0, 1) x (1, 0, 0) in component "Battery_Holder"
  circle A0 centre (-34, -30) radius 1.45
  circle A1 centre (34, -30) radius 1.45
  circle A2 centre (-34, -46) radius 1.45
  circle A3 centre (34, -46) radius 1.45
extrude "Extrude5'''''" cut sketch "Holder_Mount_Holes" along normal blind 9 from surface at 31.6 bodies 22 in component "Battery_Holder"
sketch "Batt_Post_BaseHoles" plane through (0, 0, 0) normal (0, 0, 1) x (1, 0, 0) in component "Base_Plate_Al"
  circle A0 centre (-34, -30) radius 1.45
  circle A1 centre (34, -30) radius 1.45
  circle A2 centre (-34, -46) radius 1.45
  circle A3 centre (34, -46) radius 1.45
extrude "Extrude13'" cut sketch "Batt_Post_BaseHoles" along normal blind 6 from surface at 1 bodies 1 in component "Base_Plate_Al"
sketch "Disconnect_Post_1_Sketch" plane through (0, 0, 0) normal (0, 0, 1) x (1, 0, 0) in component "Disconnect_Post_1"
  circle A0 centre (32.5, -70) radius 3
extrude "Extrude1''''''''''''''''''''''''''" add sketch "Disconnect_Post_1_Sketch" along normal blind 40 from surface at 5 separate body makes body 32 in component "Disconnect_Post_1"
sketch "PilotTop_Disconnect_Post_1" plane through (0, 0, 0) normal (0, 0, 1) x (1, 0, 0) in component "Disconnect_Post_1"
  circle A0 centre (32.5, -70) radius 1.05
extrude "Extrude2'''''''''''''''''''''" cut sketch "PilotTop_Disconnect_Post_1" against normal blind 8 from surface at 45 bodies 32 in component "Disconnect_Post_1"
sketch "PilotBot_Disconnect_Post_1" plane through (0, 0, 0) normal (0, 0, 1) x (1, 0, 0) in component "Disconnect_Post_1"
  circle A0 centre (32.5, -70) radius 1.05
extrude "Extrude3'''''''''''" cut sketch "PilotBot_Disconnect_Post_1" along normal blind 8 from surface at 5 bodies 32 in component "Disconnect_Post_1"
sketch "Disconnect_Post_2_Sketch" plane through (0, 0, 0) normal (0, 0, 1) x (1, 0, 0) in component "Disconnect_Post_2"
  circle A0 centre (51.5, -70) radius 3
extrude "Extrude1'''''''''''''''''''''''''''" add sketch "Disconnect_Post_2_Sketch" along normal blind 40 from surface at 5 separate body makes body 33 in component "Disconnect_Post_2"
sketch "PilotTop_Disconnect_Post_2" plane through (0, 0, 0) normal (0, 0, 1) x (1, 0, 0) in component "Disconnect_Post_2"
  circle A0 centre (51.5, -70) radius 1.05
extrude "Extrude2''''''''''''''''''''''" cut sketch "PilotTop_Disconnect_Post_2" against normal blind 8 from surface at 45 bodies 33 in component "Disconnect_Post_2"
sketch "PilotBot_Disconnect_Post_2" plane through (0, 0, 0) normal (0, 0, 1) x (1, 0, 0) in component "Disconnect_Post_2"
  circle A0 centre (51.5, -70) radius 1.05
extrude "Extrude3''''''''''''" cut sketch "PilotBot_Disconnect_Post_2" along normal blind 8 from surface at 5 bodies 33 in component "Disconnect_Post_2"
sketch "Disconnect_Post_BaseHoles" plane through (0, 0, 0) normal (0, 0, 1) x (1, 0, 0) in component "Base_Plate_Al"
  circle A0 centre (32.5, -70) radius 1.45
  circle A1 centre (51.5, -70) radius 1.45
extrude "Extrude14" cut sketch "Disconnect_Post_BaseHoles" along normal blind 6 from surface at 1 bodies 1 in component "Base_Plate_Al"
sketch "Disconnect_Access_Hole" plane through (0, 0, 0) normal (0, 0, 1) x (1, 0, 0) in component "Top_Cover"
  line L0 (32, -78) -> (52, -78)
  line L1 (52, -78) -> (52, -62)
  line L2 (52, -62) -> (32, -62)
  line L3 (32, -62) -> (32, -78)
extrude "Extrude6''''''" cut sketch "Disconnect_Access_Hole" along normal blind 6 from surface at 81 bodies 6 in component "Top_Cover"
sketch "PanelTap_20" plane through (0, 0, 0) normal (0, 1, 0) x (1, 0, 0) in component "Standoffs_Fasteners"
  circle A0 centre (75, -20) radius 1.25
extrude "Extrude14'" cut sketch "PanelTap_20" along normal mid plane 400 bodies 19 in component "Standoffs_Fasteners"
sketch "PanelTap_55" plane through (0, 0, 0) normal (0, 1, 0) x (1, 0, 0) in component "Standoffs_Fasteners"
  circle A0 centre (75, -55) radius 1.25
extrude "Extrude15" cut sketch "PanelTap_55" along normal mid plane 400 bodies 19 in component "Standoffs_Fasteners"
sketch "Rear_Panel_Sketch" plane through (0, 0, 0) normal (0, 0, 1) x (1, 0, 0) in component "Rear_Panel"
  line L0 (-78, -90) -> (78, -90)
  line L1 (78, -90) -> (78, -88)
  line L2 (78, -88) -> (-78, -88)
  line L3 (-78, -88) -> (-78, -90)
extrude "Extrude1''''''''''''''''''''''''''''" add sketch "Rear_Panel_Sketch" along normal blind 78 from surface at 5 separate body makes body 34 in component "Rear_Panel"
sketch "PanelClr_75_20" plane through (0, 0, 0) normal (0, 1, 0) x (1, 0, 0) in component "Rear_Panel"
  circle A0 centre (75, -20) radius 1.7
extrude "Extrude2'''''''''''''''''''''''" cut sketch "PanelClr_75_20" along normal mid plane 400 bodies 34 in component "Rear_Panel"
sketch "PanelClr_75_55" plane through (0, 0, 0) normal (0, 1, 0) x (1, 0, 0) in component "Rear_Panel"
  circle A0 centre (75, -55) radius 1.7
extrude "Extrude3'''''''''''''" cut sketch "PanelClr_75_55" along normal mid plane 400 bodies 34 in component "Rear_Panel"
sketch "PanelClr_-75_20" plane through (0, 0, 0) normal (0, 1, 0) x (1, 0, 0) in component "Rear_Panel"
  circle A0 centre (-75, -20) radius 1.7
extrude "Extrude4'''''''''" cut sketch "PanelClr_-75_20" along normal mid plane 400 bodies 34 in component "Rear_Panel"
sketch "PanelClr_-75_55" plane through (0, 0, 0) normal (0, 1, 0) x (1, 0, 0) in component "Rear_Panel"
  circle A0 centre (-75, -55) radius 1.7
extrude "Extrude5''''''" cut sketch "PanelClr_-75_55" along normal mid plane 400 bodies 34 in component "Rear_Panel"
sketch "Wedge_Pocket" plane through (0, 0, 0) normal (1, 0, 0) x (0, 0, -1) in component "Front_Wedge_L"
  line L0 (-7.5, 42.5) -> (-7.5, 85.4279)
  line L1 (-7.5, 85.4279) -> (-74.4675, 42.5)
  line L2 (-74.4675, 42.5) -> (-7.5, 42.5)
extrude "Extrude3''''''''''''''" cut sketch "Wedge_Pocket" against normal blind 42.5 from surface at -35 bodies 12 in component "Front_Wedge_L"
sketch "Wedge_HoldDown_Tap" plane through (0, 0, 0) normal (0, 0, 1) x (1, 0, 0) in component "Front_Wedge_L"
  circle A0 centre (-73, 80) radius 1.25
  circle A1 centre (-50, 50) radius 1.25
extrude "Extrude4''''''''''" cut sketch "Wedge_HoldDown_Tap" along normal blind 10 from surface at 5 bodies 12 in component "Front_Wedge_L"
sketch "Wedge_Pocket (2)" plane through (0, 0, 0) normal (1, 0, 0) x (0, 0, -1) in component "Front_Wedge_R"
  line L0 (-7.5, 42.5) -> (-7.5, 85.4279)
  line L1 (-7.5, 85.4279) -> (-74.4675, 42.5)
  line L2 (-74.4675, 42.5) -> (-7.5, 42.5)
extrude "Extrude3'''''''''''''''" cut sketch "Wedge_Pocket (2)" along normal blind 42.5 from surface at 35 bodies 13 in component "Front_Wedge_R"
sketch "Wedge_HoldDown_Tap (2)" plane through (0, 0, 0) normal (0, 0, 1) x (1, 0, 0) in component "Front_Wedge_R"
  circle A0 centre (50, 50) radius 1.25
  circle A1 centre (73, 80) radius 1.25